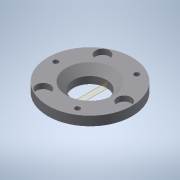
# Autodesk Inventor part: 01_SMLM_Holder_Base
Saved by Autodesk Inventor 2022 (Build 260153000, 153)
## iProperties
Created: 2021-11-24
Part Number: 01_SMLM_Holder_Base
Material: Generisch
Document SubType Name: Modeling
Designer: Muriel
Density: 1 g/cm^3
Appearance: Vorgabe
Author: Muriel
Autodesk Inventor part; units mm, degrees
ref_plane "YZ Plane" through (0, 0, 0) normal (1, 0, 0) x (0, 1, 0)
ref_plane "XZ Plane" through (0, 0, 0) normal (0, 1, 0) x (-1, 0, 0)
ref_plane "XY Plane" through (0, 0, 0) normal (0, 0, 1) x (1, 0, 0)
ref_plane "Arbeitsebene1" through (20.8918, -10.7106, -13.7095) normal (1, 0, 0) x (0, 1, 0)
sketch "Skizze1" plane through (20.8918, -10.7106, -13.7095) normal (1, 0, 0) x (0, 1, 0)
  circle A0 centre (0.052, 12) radius 1.5 construction
  line L0 (13.1827, 0) -> (-4.1221, 0)
  line L1 (-1.248, 10.5) -> (1.552, 10.5)
  line L2 (1.552, 10.5) -> (1.552, 13.5)
  line L3 (1.552, 13.5) -> (-1.048, 13.5)
  line L4 (1.552, 23.9428) -> (6.752, 23.9428)
  line L5 (6.752, 23.9428) -> (6.752, 13.5)
  line L6 (2.752, 9.5) -> (-1.248, 9.5)
  line L7 (-1.248, 9.5) -> (-1.248, 10.5)
  line L8 (6.752, 13.5) -> (2.752, 9.5)
  line L9 (-1.048, 13.5) -> (-1.048, 14.7029)
  line L10 (1.05, -14.9922) -> (1.05, 14.9922) construction
  line L11 (-1.4, -14.9922) -> (-1.4, 14.9922) construction
  line L12 (1.05, 14.9029) -> (-1.4, 14.9029) construction
  line L13 (-1.048, 14.7029) -> (1.552, 14.7029)
  line L14 (1.552, 14.7029) -> (1.552, 23.9428)
  line L15 (-2.25, 23.9428) -> (1.15, 23.9428)
  point P0 (10.7106, 13.7095)
  point P1 (6.752, 9.5)
  point P2 (-1.048, 14.9029)
  dimension "d0" = 3
  dimension "d1" = 12
  dimension "d4" = 4
  dimension "d5" = 4
  dimension "d6" = 1
  dimension "d7" = 1.3
  dimension "d8" = 2.6
  dimension "d10" = 4
  dimension "d11" = 0.2
  dimension "d20" = 0
  constraints: 26 end point, 8 perpendicular, 3 horizontal, 3 tangent, 2 point on line, 1 centre point, 8 other
  measures "d0" diameter of A0
  measures "d1" distance from line of L0 A0.centre
  measures "d4" distance of L5.end point (6.752, 9.5)
  measures "d5" distance of L6.start point (6.752, 9.5)
  measures "d6" distance between parallel lines of L6 L1
  measures "d7" distance from line of A0.centre L7
  measures "d8" distance between parallel lines of L2 L9
  measures "d10" distance from line of L7 L6.start
  measures "d20" distance between parallel lines of L15 L4
revolve "Umdrehung1" add sketch "Skizze1" angle 360 about axis through (20.8918, 2.4721, -13.7095) along (0, -1, 0)
sketch "Skizze2" plane through (20.8918, -9.1586, -13.7095) normal (0, -1, 0) x (1, 0, 0)
  circle A0 centre (9.7461, 16.8807) radius 4 projected
  circle A1 centre (-19.4922, 0) radius 4 projected
  circle A2 centre (9.7461, -16.8807) radius 4 projected
  point P0 (-20.8918, 13.7095)
hole "Bohrung1" at (30.6379, -9.1586, 3.1712) at (30.6379, -9.1586, -30.5903) at (1.3996, -9.1586, -13.7095) direction (0, 1, 0) diameter 2.9 depth 12 tip angle 118 counterbore diameter 6 counterbore depth 3
sketch "Skizze3" plane through (20.8918, -3.9586, -13.7095) normal (0, 1, 0) x (1, 0, 0)
  circle A0 centre (0, 0) radius 13.5 projected
  circle A1 centre (9.7461, -16.8807) radius 1.45 projected
  circle A2 centre (0, 0) radius 19.4922 construction
  line L0 (-9.7461, -16.8807) -> (-9.7461, 16.8807) construction
  line L1 (-9.7461, 16.8807) -> (19.4922, 0) construction
  line L2 (19.4922, 0) -> (-9.7461, -16.8807) construction
  circle A3 centre (-9.7461, -16.8807) radius 4
  circle A4 centre (-9.7461, 16.8807) radius 4
  circle A5 centre (19.4922, 0) radius 4
  point P0 (-20.8918, -13.7095)
  dimension "d21" = 8
  dimension "d22" = 8
  dimension "d23" = 8
  constraints: 6 end point, 5 coincident, 4 centre point, 2 point on circle, 7 other
  measures "d21" diameter of A3
  measures "d22" diameter of A4
  measures "d23" diameter of A5
extrude "Extrusion1" cut sketch "Skizze3" against normal blind 3 contours A3 | A4 | A5
sketch "Skizze4" plane through (20.8918, -9.1586, -13.7095) normal (0, -1, 0) x (1, 0, 0)
  circle A0 centre (0, 0) radius 13.5 projected
  circle A1 centre (0, 0) radius 10.5 projected
  point P0 (-20.8918, 13.7095)
extrude "Extrusion2" add sketch "Skizze4" along normal blind 0.5
equation "\"d5\" = d4"
